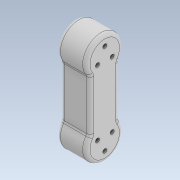
# Autodesk Inventor part: thigh
Saved by Autodesk Inventor 2020 (Build 240168000, 168)
## iProperties
Created: 2020-12-24
Part Number: thigh
Material: Generic
Document SubType Name: Modeling
Designer: DELL
Density: 1 g/cm^3
Appearance: Default
Author: DELL
Autodesk Inventor part; units mm, degrees
ref_plane "YZ Plane" through (0, 0, 0) normal (1, 0, 0) x (0, 1, 0)
ref_plane "XZ Plane" through (0, 0, 0) normal (0, 1, 0) x (-1, 0, 0)
sketch "Sketch1" plane through (0, 0, 0) normal (1, 0, 0) x (0, 1, 0)
  arc A0 (-15, -20) -> (-15, 20) centre (0, 0) ccw
  line L0 (-15, 20) -> (-50, 20)
  line L1 (-15, -20) -> (-50, -20)
  circle A1 centre (0, 0) radius 11.5 construction
  line L2 (25, 0) -> (0, 0) construction
  line L3 (0, 0) -> (-7.125, 12.3409) construction
  line L4 (0, 0) -> (-7.125, -12.3409) construction
  line L5 (-15, 20) -> (-15, -20) construction
  circle A2 centre (11.5, 0) radius 1.65
  circle A3 centre (-5.75, 9.9593) radius 1.65
  circle A4 centre (-5.75, -9.9593) radius 1.65
  circle A5 centre (11.5, 0) radius 2.75
  circle A6 centre (-5.75, -9.9593) radius 2.75
  circle A7 centre (-5.75, 9.9593) radius 2.75
  line L6 (0, 0) -> (5.8575, 10.1455) construction
  line L7 (0, 0) -> (5.8575, -10.1455) construction
  circle A8 centre (0, 0) radius 9.715 construction
  circle A9 centre (4.8575, 8.4134) radius 2
  circle A10 centre (4.8575, -8.4134) radius 2
  circle A11 centre (-9.715, 0) radius 2
  line L8 (-50, 20) -> (-50, -20) construction
  line L9 (-50, -20) -> (-50, 20)
  line L10 (0, 25) -> (0, -25) construction
  point P0 (-15, 0)
  dimension "d6" = 4
  dimension "d0" = 23
  dimension "d1" = 30
  dimension "d2" = 3.3
  dimension "d3" = 5.5
  dimension "d4" = 30
  dimension "d5" = 19.43
  dimension "d7" = 50
  dimension "d18" = 50
  dimension "d19" = 40
  constraints: 22 end point, 11 point on circle, 8 centre point, 6 coincident, 5 point on line, 3 vertical, 2 equal length, 2 equal radius, 2 horizontal, 2 midpoint, 1 horizontal alignment, 16 other
  measures "d0" diameter of A1
  measures "d1" angle of L3 L5
  measures "d2" diameter of A2
  measures "d3" diameter of A5
  measures "d4" angle of L5 L6
  measures "d5" diameter of A8
  measures "d7" diameter of A0
  measures "d18" distance between parallel lines of L8 L10
  measures "d19" distance between parallel lines of L1 L0
extrude "Extrusion1" add sketch "Sketch1" along normal mid plane 40 contours L1 L9 L0 A0 | A5 | A6 | A7 | A9 | A10 | A11
extrude "Extrusion2" cut sketch "Sketch1" against normal blind 35 from surface at 20 contours A5 | A6 | A7
extrude "Extrusion3" cut sketch "Sketch1" along normal blind 5 from surface at -20 contours A9 | A10 | A11
ref_plane "Work Plane1" through (0, -50, 20) normal (0, -1, 0) x (0, 0, -1)
mirror "Mirror1" about plane through (0, -50, 20) normal (0, -1, 0)
fillet "Fillet1" radius 5 12 edges at (-20, -125, 0) (-20, -50, -20) (-20, 25, 0) (-20, -50, 20) (20, -125, 0) (20, -50, -20) (20, 25, 0) (20, -50, 20) (0, -15, 20) (0, -85, 20) (0, -85, -20) (0, -15, -20)
equation "\"d18\" = 0.5 * thigh_length"
equation "\"thigh_length\" = 100"
body "Solid1"
